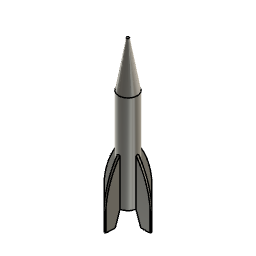
auk3 v2 (Autodesk Fusion 360 design; units mm, degrees)
Autodesk Fusion 360 part; units mm, degrees
sketch "Sketch1" plane through (0, 0, 0) normal (0, 0, 1) x (1, 0, 0)
  circle A0 centre (0, 0) radius 14
  circle A1 centre (0, 0) radius 20
  line L0 (-19.8298, 2.6034) -> (-49.02, 2.0196)
  line L1 (-19.8298, -2.6034) -> (-49.02, -2.0196)
  line L2 (-50, 1.0198) -> (-50, -1.0198)
  arc A2 (-49.02, 2.0196) -> (-50, 1.0198) centre (-49, 1.0198) ccw
  arc A3 (-50, -1.0198) -> (-49.02, -2.0196) centre (-49, -1.0198) ccw
  line L3 (-2.6034, -19.8298) -> (-2.0196, -49.02)
  line L4 (-1.0198, -50) -> (1.0198, -50)
  arc A4 (-2.0196, -49.02) -> (-1.0198, -50) centre (-1.0198, -49) ccw
  arc A5 (1.0198, -50) -> (2.0196, -49.02) centre (1.0198, -49) ccw
  line L5 (2.6034, -19.8298) -> (2.0196, -49.02)
  line L6 (19.8298, -2.6034) -> (49.02, -2.0196)
  line L7 (50, -1.0198) -> (50, 1.0198)
  arc A6 (49.02, -2.0196) -> (50, -1.0198) centre (49, -1.0198) ccw
  arc A7 (50, 1.0198) -> (49.02, 2.0196) centre (49, 1.0198) ccw
  line L8 (19.8298, 2.6034) -> (49.02, 2.0196)
  line L9 (2.6034, 19.8298) -> (2.0196, 49.02)
  line L10 (1.0198, 50) -> (-1.0198, 50)
  arc A8 (2.0196, 49.02) -> (1.0198, 50) centre (1.0198, 49) ccw
  arc A9 (-1.0198, 50) -> (-2.0196, 49.02) centre (-1.0198, 49) ccw
  line L11 (-2.6034, 19.8298) -> (-2.0196, 49.02)
  dimension "d1" = 28
  dimension "d2" = 40
  dimension "d3" = 1
  dimension "d5" = 360
  constraint coincident A0.centre A1.centre
  constraint concentric A0 A1
  constraint vertical L2
  constraint coincident A1 L0.start
  constraint coincident A1 L1.start
  constraint tangent L0 A2
  constraint tangent L2 A2
  constraint tangent L1 A3
  constraint tangent L2 A3
  constraint equal A2 A3
  measures "d1" diameter of A0
  measures "d2" diameter of A1
  measures "d3" radius of A2
extrude "Extrude1" add sketch "Sketch1" along normal blind 130
extrude "Extrude2" cut sketch "Sketch1" along normal blind 30 contours A1
sketch "Sketch2" plane through (0, 0, 130) normal (0, 0, 1) x (-1, 0, 0)
  circle A0 centre (0, 0) radius 14
  line L0 (19.8298, -2.6034) -> (49.02, -2.0196)
  arc A1 (49.02, -2.0196) -> (50, -1.0198) centre (49, -1.0198) ccw
  line L1 (50, -1.0198) -> (50, 1.0198)
  arc A2 (50, 1.0198) -> (49.02, 2.0196) centre (49, 1.0198) ccw
  line L2 (49.02, 2.0196) -> (19.8298, 2.6034)
  arc A3 (19.8298, 2.6034) -> (2.6034, 19.8298) centre (0, 0) ccw
  line L3 (2.6034, 19.8298) -> (2.0196, 49.02)
  arc A4 (2.0196, 49.02) -> (1.0198, 50) centre (1.0198, 49) ccw
  line L4 (1.0198, 50) -> (-1.0198, 50)
  arc A5 (-1.0198, 50) -> (-2.0196, 49.02) centre (-1.0198, 49) ccw
  line L5 (-2.0196, 49.02) -> (-2.6034, 19.8298)
  arc A6 (-2.6034, 19.8298) -> (-19.8298, 2.6034) centre (0, 0) ccw
  line L6 (-19.8298, 2.6034) -> (-49.02, 2.0196)
  arc A7 (-49.02, 2.0196) -> (-50, 1.0198) centre (-49, 1.0198) ccw
  line L7 (-50, 1.0198) -> (-50, -1.0198)
  arc A8 (-50, -1.0198) -> (-49.02, -2.0196) centre (-49, -1.0198) ccw
  line L8 (-49.02, -2.0196) -> (-19.8298, -2.6034)
  arc A9 (-19.8298, -2.6034) -> (-2.6034, -19.8298) centre (0, 0) ccw
  line L9 (-2.6034, -19.8298) -> (-2.0196, -49.02)
  arc A10 (-2.0196, -49.02) -> (-1.0198, -50) centre (-1.0198, -49) ccw
  line L10 (-1.0198, -50) -> (1.0198, -50)
  arc A11 (1.0198, -50) -> (2.0196, -49.02) centre (1.0198, -49) ccw
  line L11 (2.0196, -49.02) -> (2.6034, -19.8298)
  arc A12 (2.6034, -19.8298) -> (19.8298, -2.6034) centre (0, 0) ccw
  circle A13 centre (0, 0) radius 14
  circle A14 centre (0, 0) radius 20
  constraint concentric A0 A13
  constraint concentric A0 A14
extrude "Extrude3" add sketch "Sketch2" along normal blind 30 contours A3 A6 A9 A12 A14
sketch "Sketch3" plane through (0, 0, 0) normal (0, 1, 0) x (1, 0, 0)
  arc A0 (20, -130) -> (50, -30) centre (-122.2891, -32.8133) ccw
  line L0 (20, -130) -> (20, -155)
  line L1 (20, -155) -> (75, -155)
  line L2 (75, -155) -> (75, -30)
  line L3 (75, -30) -> (50, -30)
  constraint vertical L0
  constraint perpendicular L0 L1
  constraint perpendicular L1 L2
  constraint perpendicular L0 L3
revolve "Revolve1" cut sketch "Sketch3" angle 360 about axis through (0, 0, 1.75) along (0, 0, 1)
sketch "Sketch4" plane through (0, 0, 0) normal (0, 1, 0) x (1, 0, 0)
  line L0 (-20, -30) -> (-30, 0)
  line L1 (-30, 0) -> (0, 0)
  line L2 (0, 0) -> (0, -30)
  line L3 (0, -30) -> (-20, -30)
  constraint coincident L1.end L2.start
  constraint horizontal L1
  constraint perpendicular L1 L2
  constraint perpendicular L2 L3
revolve "Revolve2" cut sketch "Sketch4" angle 360 about axis through (0, 0, 0) along (0, 0, 1)
sketch "Sketch5" plane through (0, 0, 160) normal (0, 0, 1) x (-1, 0, 0)
  circle A0 centre (0, 0) radius 14
  circle A1 centre (0, 0) radius 20
  circle A2 centre (0, 0) radius 20
  constraint concentric A0 A2
extrude "Extrude4" add sketch "Sketch5" along normal blind 80 contours A0 | A1 A2
extrude "Extrude5" add 1 faces at (-6.9042, -3.3249, 240) along direction (0, 0, 1) blind 100 draft -10
fillet "Fillet1" radius 2 1 edges at (2.2071, -0.8561, 340)
